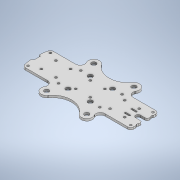
# Autodesk Inventor part: center plate
Saved by Autodesk Inventor 2020 (Build 240168000, 168)
## iProperties
Created: 2022-08-17
Part Number: center plate
Material: Generic
Document SubType Name: Modeling
Designer: Steven
Density: 1 g/cm^3
Appearance: Default
Author: Steven
Autodesk Inventor part; units mm, degrees
ref_plane "YZ Plane" through (0, 0, 0) normal (1, 0, 0) x (0, 1, 0)
ref_plane "XZ Plane" through (0, 0, 0) normal (0, 1, 0) x (-1, 0, 0)
ref_plane "XY Plane" through (0, 0, 0) normal (0, 0, 1) x (1, 0, 0)
sketch "Sketch1" plane through (0, 0, 0) normal (0, 1, 0) x (-1, 0, 0)
  arc A0 (-33.8239, -28.265) -> (-21.4136, -36.6803) centre (-27.5042, -32.3038) ccw
  line L0 (-21.4136, -36.6803) -> (-21.3077, -36.5329)
  arc A1 (21.3077, -36.5329) -> (-21.3077, -36.5329) centre (0, -51.9445) ccw
  line L1 (21.3077, -36.5329) -> (21.4136, -36.6803)
  arc A2 (21.4136, -36.6803) -> (33.8239, -28.265) centre (27.5042, -32.3038) ccw
  arc A3 (33.327, -27.1322) -> (33.8239, -28.265) centre (37.1944, -26.111) ccw
  arc A4 (39.3981, -19.25) -> (33.327, -27.1322) centre (39.3981, -25.5292) ccw
  line L2 (39.3981, -19.25) -> (69.95, -19.25)
  arc A5 (69.95, -19.25) -> (73.8582, -16.102) centre (69.95, -15.25) ccw
  arc A6 (73.8582, -16.102) -> (75.3578, -5.9597) centre (0.0002, 0) ccw
  arc A7 (75.3578, -5.9597) -> (74.448, -4.8846) centre (74.3609, -5.8808) ccw
  line L3 (74.448, -4.8846) -> (73.7452, -4.8231)
  arc A8 (72.8337, -3.7752) -> (73.7452, -4.8231) centre (73.8323, -3.8269) ccw
  arc A9 (72.8337, -3.7752) -> (72.8337, 3.7752) centre (0.0002, 0) ccw
  arc A10 (73.7452, 4.8231) -> (72.8337, 3.7752) centre (73.8323, 3.8269) ccw
  line L4 (73.7452, 4.8231) -> (74.448, 4.8846)
  arc A11 (74.448, 4.8846) -> (75.3578, 5.9597) centre (74.3609, 5.8808) ccw
  arc A12 (75.3578, 5.9597) -> (73.8582, 16.102) centre (0.0002, 0) ccw
  arc A13 (73.8582, 16.102) -> (69.95, 19.25) centre (69.95, 15.25) ccw
  line L5 (69.95, 19.25) -> (39.3981, 19.25)
  arc A14 (33.327, 27.1322) -> (39.3981, 19.25) centre (39.3981, 25.5292) ccw
  arc A15 (33.8239, 28.265) -> (33.327, 27.1322) centre (37.1944, 26.111) ccw
  arc A16 (33.8239, 28.265) -> (21.4136, 36.6803) centre (27.5042, 32.3038) ccw
  line L6 (21.4136, 36.6803) -> (21.3077, 36.5329)
  arc A17 (-21.3077, 36.5329) -> (21.3077, 36.5329) centre (0, 51.9445) ccw
  line L7 (-21.3077, 36.5329) -> (-21.4136, 36.6803)
  arc A18 (-21.4136, 36.6803) -> (-33.8239, 28.265) centre (-27.5042, 32.3038) ccw
  arc A19 (-33.327, 27.1322) -> (-33.8239, 28.265) centre (-37.1944, 26.111) ccw
  arc A20 (-39.3981, 19.25) -> (-33.327, 27.1322) centre (-39.3981, 25.5292) ccw
  line L8 (-39.3981, 19.25) -> (-70.5602, 19.25)
  arc A21 (-70.5602, 19.25) -> (-74.56, 15.2108) centre (-70.5602, 15.25) ccw
  line L9 (-74.56, 15.2108) -> (-74.56, 12.5073)
  arc A22 (-74.56, 12.5073) -> (-74.0519, 11.382) centre (-73.06, 12.5073) ccw
  arc A23 (-73.6342, 9.7438) -> (-74.0519, 11.382) centre (-75.0438, 10.2568) ccw
  line L10 (-73.6342, 9.7438) -> (-74.2404, 8.0784)
  arc A24 (-74.2404, 8.0784) -> (-74.56, 6.2657) centre (-69.26, 6.2657) ccw
  line L11 (-74.56, 6.2657) -> (-74.56, 6.25)
  arc A25 (-74.56, 6.25) -> (-71.56, 3.25) centre (-71.56, 6.25) ccw
  line L12 (-71.56, 3.25) -> (-65.309, 3.25)
  arc A26 (-65.309, -3.25) -> (-65.309, 3.25) centre (-65.309, 0) ccw
  line L13 (-65.309, -3.25) -> (-71.56, -3.25)
  arc A27 (-71.56, -3.25) -> (-74.56, -6.25) centre (-71.56, -6.25) ccw
  line L14 (-74.56, -6.25) -> (-74.56, -6.2657)
  arc A28 (-74.56, -6.2657) -> (-74.2404, -8.0784) centre (-69.26, -6.2657) ccw
  line L15 (-74.2404, -8.0784) -> (-73.6342, -9.7438)
  arc A29 (-74.0519, -11.382) -> (-73.6342, -9.7438) centre (-75.0438, -10.2568) ccw
  arc A30 (-74.0519, -11.382) -> (-74.56, -12.5073) centre (-73.06, -12.5073) ccw
  line L16 (-74.56, -12.5073) -> (-74.56, -15.2108)
  arc A31 (-74.56, -15.2108) -> (-70.5602, -19.25) centre (-70.5602, -15.25) ccw
  line L17 (-70.5602, -19.25) -> (-39.3981, -19.25)
  arc A32 (-33.327, -27.1322) -> (-39.3981, -19.25) centre (-39.3981, -25.5292) ccw
  arc A33 (-33.8239, -28.265) -> (-33.327, -27.1322) centre (-37.1944, -26.111) ccw
  circle A34 centre (-27.5042, -32.3038) radius 2.25
  arc A35 (-8.7852, -24.3068) -> (-9.9324, -22.6685) centre (-9.3588, -23.4876) ccw
  line L18 (-11.9802, -24.1024) -> (-9.9324, -22.6685)
  line L19 (58.6187, 4.75) -> (65.1187, 4.75)
  arc A36 (65.1187, 4.75) -> (65.1187, 7.75) centre (65.1187, 6.25) ccw
  line L20 (65.1187, 7.75) -> (58.6187, 7.75)
  arc A37 (58.6187, 7.75) -> (58.6187, 4.75) centre (58.6187, 6.25) ccw
  line L21 (-18.0988, -21.6995) -> (-22.3003, -27.5465)
  arc A38 (-24.6553, -25.8542) -> (-22.3003, -27.5465) centre (-23.4778, -26.7004) ccw
  circle A39 centre (27.5042, -32.3038) radius 3.15
  arc A40 (-18.0988, -21.6995) -> (-20.4538, -20.0072) centre (-19.2763, -20.8534) ccw
  line L22 (65.1187, 1.5) -> (56.2002, 1.5)
  arc A41 (56.2002, 1.5) -> (56.2002, -1.5) centre (56.2002, 0) ccw
  line L23 (56.2002, -1.5) -> (65.1187, -1.5)
  arc A42 (65.1187, -1.5) -> (65.1187, 1.5) centre (65.1187, 0) ccw
  line L24 (30.3675, -6.2794) -> (31.6059, -1.9507)
  arc A43 (33.0971, -1.3777) -> (31.6059, -1.9507) centre (32.5673, -2.2258) ccw
  line L25 (33.0971, -1.3777) -> (38.3837, -4.6803)
  arc A44 (38.0092, -6.5163) -> (38.3837, -4.6803) centre (37.8539, -5.5284) ccw
  line L26 (38.0092, -6.5163) -> (31.4843, -7.5423)
  arc A45 (30.3675, -6.2794) -> (31.4843, -7.5423) centre (31.329, -6.5544) ccw
  arc A46 (-11.9802, -24.1024) -> (-10.8331, -25.7407) centre (-11.4067, -24.9216) ccw
  circle A47 centre (-27.5042, -32.3038) radius 3.15
  line L27 (44.5187, 14.25) -> (53.5187, 14.25)
  arc A48 (53.5187, 14.25) -> (54.5187, 14.25) centre (54.0187, 14.25) ccw
  line L28 (54.5187, 14.25) -> (54.5187, 16.25)
  arc A49 (54.5187, 16.25) -> (53.5187, 16.25) centre (54.0187, 16.25) ccw
  line L29 (53.5187, 16.25) -> (44.5187, 16.25)
  arc A50 (44.5187, 16.25) -> (43.5187, 16.25) centre (44.0187, 16.25) ccw
  line L30 (43.5187, 16.25) -> (43.5187, 14.25)
  arc A51 (43.5187, 14.25) -> (44.5187, 14.25) centre (44.0187, 14.25) ccw
  line L31 (-8.7852, -24.3068) -> (-10.8331, -25.7407)
  circle A52 centre (57.0593, 10) radius 1
  arc A53 (-22.3003, 27.5465) -> (-24.6553, 25.8542) centre (-23.4778, 26.7004) ccw
  circle A54 centre (69.95, 15.25) radius 1.55
  line L32 (-9.9324, 22.6685) -> (-11.9802, 24.1024)
  line L33 (-70.7795, -9.0168) -> (-71.6345, -6.6675)
  arc A55 (-71.6345, -6.6675) -> (-72.2754, -6.3687) centre (-72.1044, -6.8386) ccw
  line L34 (-72.2754, -6.3687) -> (-72.7452, -6.5397)
  arc A56 (-72.7452, -6.5397) -> (-73.044, -7.1806) centre (-72.5742, -7.0096) ccw
  line L35 (-73.044, -7.1806) -> (-72.189, -9.5298)
  arc A57 (-72.189, -9.5298) -> (-71.5481, -9.8286) centre (-71.7192, -9.3588) ccw
  line L36 (-71.5481, -9.8286) -> (-71.0783, -9.6576)
  arc A58 (-71.0783, -9.6576) -> (-70.7795, -9.0168) centre (-71.2493, -9.1878) ccw
  circle A59 centre (-9.9998, 10) radius 1.55
  circle A60 centre (-28.2498, 15.25) radius 1.55
  arc A61 (-38.0092, 6.5163) -> (-38.3837, 4.6803) centre (-37.8539, 5.5284) ccw
  line L37 (-38.0092, 6.5163) -> (-31.4843, 7.5423)
  arc A62 (-30.3675, 6.2794) -> (-31.4843, 7.5423) centre (-31.329, 6.5544) ccw
  line L38 (-30.3675, 6.2794) -> (-31.6059, 1.9507)
  arc A63 (-33.0971, 1.3777) -> (-31.6059, 1.9507) centre (-32.5673, 2.2258) ccw
  line L39 (-33.0971, 1.3777) -> (-38.3837, 4.6803)
  line L40 (-42.405, -16.5) -> (-62.405, -16.5)
  arc A64 (-62.405, -14.5) -> (-62.405, -16.5) centre (-62.405, -15.5) ccw
  line L41 (-62.405, -14.5) -> (-42.405, -14.5)
  arc A65 (-42.405, -16.5) -> (-42.405, -14.5) centre (-42.405, -15.5) ccw
  line L42 (-71.0783, 9.6576) -> (-71.5481, 9.8286)
  arc A66 (-71.5481, 9.8286) -> (-72.189, 9.5298) centre (-71.7192, 9.3588) ccw
  line L43 (-72.189, 9.5298) -> (-73.044, 7.1806)
  arc A67 (-73.044, 7.1806) -> (-72.7452, 6.5397) centre (-72.5742, 7.0096) ccw
  line L44 (-72.7452, 6.5397) -> (-72.2754, 6.3687)
  arc A68 (-72.2754, 6.3687) -> (-71.6345, 6.6675) centre (-72.1044, 6.8386) ccw
  line L45 (-71.6345, 6.6675) -> (-70.7795, 9.0168)
  arc A69 (-70.7795, 9.0168) -> (-71.0783, 9.6576) centre (-71.2493, 9.1878) ccw
  arc A70 (-58.3158, -3.5) -> (-58.3158, -5.5) centre (-58.3158, -4.5) ccw
  line L46 (-58.3158, -5.5) -> (-52.3158, -5.5)
  arc A71 (-52.3158, -5.5) -> (-52.3158, -3.5) centre (-52.3158, -4.5) ccw
  line L47 (-52.3158, -3.5) -> (-58.3158, -3.5)
  line L48 (-10.8331, 25.7407) -> (-8.7852, 24.3068)
  arc A72 (-20.4275, 8.2673) -> (-20.8836, 6.6042) centre (-20.4038, 7.3667) ccw
  line L49 (-20.4275, 8.2673) -> (-13.542, 8.3985)
  arc A73 (-12.661, 7.2587) -> (-13.542, 8.3985) centre (-13.5284, 7.4986) ccw
  line L50 (-12.661, 7.2587) -> (-13.6696, 3.6122)
  arc A74 (-15.1632, 3.0306) -> (-13.6696, 3.6122) centre (-14.6334, 3.8788) ccw
  line L51 (-15.1632, 3.0306) -> (-20.8836, 6.6042)
  arc A75 (-20.4538, 20.0072) -> (-18.0988, 21.6995) centre (-19.2763, 20.8534) ccw
  arc A76 (-10.8331, 25.7407) -> (-11.9802, 24.1024) centre (-11.4067, 24.9216) ccw
  circle A77 centre (-57.059, 10) radius 1.55
  arc A78 (-58.3158, 5.5) -> (-58.3158, 3.5) centre (-58.3158, 4.5) ccw
  line L52 (-58.3158, 3.5) -> (-52.3158, 3.5)
  arc A79 (-52.3158, 3.5) -> (-52.3158, 5.5) centre (-52.3158, 4.5) ccw
  line L53 (-52.3158, 5.5) -> (-58.3158, 5.5)
  line L54 (-24.6553, 25.8542) -> (-20.4538, 20.0072)
  arc A80 (-9.9324, 22.6685) -> (-8.7852, 24.3068) centre (-9.3588, 23.4876) ccw
  circle A81 centre (-15.25, 15.25) radius 2.25
  line L55 (-62.405, 16.5) -> (-42.405, 16.5)
  arc A82 (-42.405, 14.5) -> (-42.405, 16.5) centre (-42.405, 15.5) ccw
  line L56 (-42.405, 14.5) -> (-62.405, 14.5)
  arc A83 (-62.405, 16.5) -> (-62.405, 14.5) centre (-62.405, 15.5) ccw
  arc A84 (-44.4091, 0.275) -> (-44.4091, -0.275) centre (-43.4477, 0) ccw
  line L57 (-44.4091, 0.275) -> (-43.6501, 2.9283)
  arc A85 (-42.1588, 3.5013) -> (-43.6501, 2.9283) centre (-42.6886, 2.6532) ccw
  line L58 (-42.1588, 3.5013) -> (-37.9117, 0.8481)
  arc A86 (-37.9117, -0.8481) -> (-37.9117, 0.8481) centre (-38.4415, 0) ccw
  line L59 (-37.9117, -0.8481) -> (-42.1588, -3.5013)
  arc A87 (-43.6501, -2.9283) -> (-42.1588, -3.5013) centre (-42.6886, -2.6532) ccw
  line L60 (-43.6501, -2.9283) -> (-44.4091, -0.275)
  arc A88 (-7.8639, 3.9177) -> (-9.3575, 3.336) centre (-8.3937, 3.0696) ccw
  line L61 (-7.8639, 3.9177) -> (-2.9502, 0.8481)
  arc A89 (-2.9502, -0.8481) -> (-2.9502, 0.8481) centre (-3.48, 0) ccw
  line L62 (-2.9502, -0.8481) -> (-7.8639, -3.9177)
  arc A90 (-9.3575, -3.336) -> (-7.8639, -3.9177) centre (-8.3937, -3.0696) ccw
  line L63 (-9.3575, -3.336) -> (-10.206, -0.2664)
  arc A91 (-10.206, 0.2664) -> (-10.206, -0.2664) centre (-9.2421, 0) ccw
  line L64 (-10.206, 0.2664) -> (-9.3575, 3.336)
  circle A92 centre (-15.25, 15.25) radius 3.15
  circle A93 centre (-37.059, 10) radius 1.55
  circle A94 centre (-70.5602, 15.25) radius 1.55
  circle A95 centre (-70.5602, -15.25) radius 1.55
  circle A96 centre (28.2502, -15.25) radius 1.55
  line L65 (22.3006, -27.5465) -> (18.0991, -21.6995)
  line L66 (10.8331, -25.7407) -> (8.7852, -24.3068)
  arc A97 (10.8331, -25.7407) -> (11.9802, -24.1024) centre (11.4067, -24.9216) ccw
  arc A98 (-0.5298, 4.0525) -> (0.5298, 4.0525) centre (0, 4.9006) ccw
  line L67 (-0.5298, 4.0525) -> (-4.9689, 6.8256)
  arc A99 (-4.4965, 8.4889) -> (-4.9689, 6.8256) centre (-4.492, 7.5889) ccw
  line L68 (-4.4965, 8.4889) -> (4.4965, 8.4889)
  arc A100 (4.9689, 6.8256) -> (4.4965, 8.4889) centre (4.492, 7.5889) ccw
  line L69 (4.9689, 6.8256) -> (0.5298, 4.0525)
  line L70 (10.206, -0.2664) -> (9.3575, -3.336)
  arc A101 (7.8639, -3.9177) -> (9.3575, -3.336) centre (8.3937, -3.0696) ccw
  line L71 (7.8639, -3.9177) -> (2.9502, -0.8481)
  arc A102 (2.9502, 0.8481) -> (2.9502, -0.8481) centre (3.48, 0) ccw
  line L72 (2.9502, 0.8481) -> (7.8639, 3.9177)
  arc A103 (9.3575, 3.336) -> (7.8639, 3.9177) centre (8.3937, 3.0696) ccw
  line L73 (9.3575, 3.336) -> (10.206, 0.2664)
  arc A104 (10.206, -0.2664) -> (10.206, 0.2664) centre (9.2421, 0) ccw
  line L74 (27.1605, 4.3044) -> (28.3132, 0.275)
  arc A105 (28.3132, -0.275) -> (28.3132, 0.275) centre (27.3517, 0) ccw
  line L75 (28.3132, -0.275) -> (27.1605, -4.3044)
  arc A106 (25.6692, -4.8775) -> (27.1605, -4.3044) centre (26.199, -4.0294) ccw
  line L76 (25.6692, -4.8775) -> (19.2192, -0.8481)
  arc A107 (19.2192, 0.8481) -> (19.2192, -0.8481) centre (19.749, 0) ccw
  line L77 (19.2192, 0.8481) -> (25.6692, 4.8775)
  arc A108 (27.1605, 4.3044) -> (25.6692, 4.8775) centre (26.199, 4.0294) ccw
  arc A109 (-4.9689, -6.8256) -> (-4.4965, -8.4889) centre (-4.492, -7.5889) ccw
  line L78 (-4.9689, -6.8256) -> (-0.5298, -4.0525)
  arc A110 (0.5298, -4.0525) -> (-0.5298, -4.0525) centre (0, -4.9006) ccw
  line L79 (0.5298, -4.0525) -> (4.9689, -6.8256)
  arc A111 (4.4965, -8.4889) -> (4.9689, -6.8256) centre (4.492, -7.5889) ccw
  line L80 (4.4965, -8.4889) -> (-4.4965, -8.4889)
  circle A112 centre (10.0002, -10) radius 1.55
  arc A113 (20.4275, -8.2673) -> (20.8836, -6.6042) centre (20.4067, -7.3675) ccw
  ellipse E0 centre (0, 0) end of major axis (87.8993, 0) minor radius 8.5 (13.542, -8.3985) -> (20.4275, -8.2673) ccw
  line L81 (12.661, -7.2587) -> (13.6696, -3.6122)
  line L82 (15.1632, -3.0306) -> (20.8836, -6.6042)
  arc A114 (13.6696, 3.6122) -> (15.1632, 3.0306) centre (14.6334, 3.8788) ccw
  arc A115 (12.661, -7.2587) -> (13.542, -8.3985) centre (13.5284, -7.4986) ccw
  arc A116 (15.1632, -3.0306) -> (13.6696, -3.6122) centre (14.6334, -3.8788) ccw
  arc A117 (20.4541, -20.0072) -> (18.0991, -21.6995) centre (19.2766, -20.8534) ccw
  arc A118 (9.9324, -22.6685) -> (8.7852, -24.3068) centre (9.3588, -23.4876) ccw
  arc A119 (22.3006, -27.5465) -> (24.6556, -25.8542) centre (23.4781, -26.7004) ccw
  circle A120 centre (15.25, -15.25) radius 2.25
  line L83 (9.9324, -22.6685) -> (11.9802, -24.1024)
  line L84 (20.4541, -20.0072) -> (24.6556, -25.8542)
  circle A121 centre (27.5042, -32.3038) radius 2.25
  circle A122 centre (37.0593, 10) radius 1
  arc A123 (44.4091, -0.275) -> (44.4091, 0.275) centre (43.4477, 0) ccw
  line L85 (44.4091, -0.275) -> (43.6501, -2.9283)
  arc A124 (42.1588, -3.5013) -> (43.6501, -2.9283) centre (42.6886, -2.6532) ccw
  line L86 (42.1588, -3.5013) -> (37.9117, -0.8481)
  arc A125 (37.9117, 0.8481) -> (37.9117, -0.8481) centre (38.4415, 0) ccw
  line L87 (37.9117, 0.8481) -> (42.1588, 3.5013)
  arc A126 (43.6501, 2.9283) -> (42.1588, 3.5013) centre (42.6886, 2.6532) ccw
  line L88 (43.6501, 2.9283) -> (44.4091, 0.275)
  line L89 (31.6059, 1.9507) -> (30.3675, 6.2794)
  arc A127 (31.4843, 7.5423) -> (30.3675, 6.2794) centre (31.329, 6.5544) ccw
  line L90 (31.4843, 7.5423) -> (38.0092, 6.5163)
  arc A128 (38.3837, 4.6803) -> (38.0092, 6.5163) centre (37.8539, 5.5284) ccw
  line L91 (38.3837, 4.6803) -> (33.0971, 1.3777)
  arc A129 (31.6059, 1.9507) -> (33.0971, 1.3777) centre (32.5673, 2.2258) ccw
  ellipse E1 centre (0, 0) end of major axis (87.8993, 0) minor radius 8.5 (20.4275, 8.2673) -> (13.542, 8.3985) ccw
  line L92 (20.8836, 6.6042) -> (15.1632, 3.0306)
  arc A130 (20.8836, 6.6042) -> (20.4275, 8.2673) centre (20.4067, 7.3675) ccw
  arc A131 (13.542, 8.3985) -> (12.661, 7.2587) centre (13.5284, 7.4986) ccw
  circle A132 centre (10.0002, 10) radius 1.55
  line L93 (13.6696, 3.6122) -> (12.661, 7.2587)
  circle A133 centre (15.25, -15.25) radius 3.15
  line L94 (24.6556, 25.8542) -> (20.4541, 20.0072)
  line L95 (43.5187, -14.25) -> (43.5187, -16.25)
  arc A134 (43.5187, -16.25) -> (44.5187, -16.25) centre (44.0187, -16.25) ccw
  line L96 (44.5187, -16.25) -> (53.5187, -16.25)
  arc A135 (53.5187, -16.25) -> (54.5187, -16.25) centre (54.0187, -16.25) ccw
  line L97 (54.5187, -16.25) -> (54.5187, -14.25)
  arc A136 (54.5187, -14.25) -> (53.5187, -14.25) centre (54.0187, -14.25) ccw
  line L98 (53.5187, -14.25) -> (44.5187, -14.25)
  arc A137 (44.5187, -14.25) -> (43.5187, -14.25) centre (44.0187, -14.25) ccw
  circle A138 centre (37.0593, -10) radius 1
  circle A139 centre (57.0593, -10) radius 1
  line L99 (58.6187, -7.75) -> (65.1187, -7.75)
  arc A140 (65.1187, -7.75) -> (65.1187, -4.75) centre (65.1187, -6.25) ccw
  line L100 (65.1187, -4.75) -> (58.6187, -4.75)
  arc A141 (58.6187, -4.75) -> (58.6187, -7.75) centre (58.6187, -6.25) ccw
  circle A142 centre (69.95, -15.25) radius 1.55
  arc A143 (8.7852, 24.3068) -> (9.9324, 22.6685) centre (9.3588, 23.4876) ccw
  arc A144 (11.9802, 24.1024) -> (10.8331, 25.7407) centre (11.4067, 24.9216) ccw
  circle A145 centre (15.25, 15.25) radius 3.15
  line L101 (11.9802, 24.1024) -> (9.9324, 22.6685)
  arc A146 (24.6556, 25.8542) -> (22.3006, 27.5465) centre (23.4781, 26.7004) ccw
  circle A147 centre (15.25, 15.25) radius 2.25
  line L102 (18.0991, 21.6995) -> (22.3006, 27.5465)
  line L103 (-18.0988, 21.6995) -> (-22.3003, 27.5465)
  line L104 (8.7852, 24.3068) -> (10.8331, 25.7407)
  circle A148 centre (28.2502, 15.25) radius 1.55
  arc A149 (18.0991, 21.6995) -> (20.4541, 20.0072) centre (19.2766, 20.8534) ccw
  arc A150 (-13.542, -8.3985) -> (-12.661, -7.2587) centre (-13.5284, -7.4986) ccw
  line L105 (-13.542, -8.3985) -> (-20.4275, -8.2673)
  arc A151 (-20.8836, -6.6042) -> (-20.4275, -8.2673) centre (-20.4067, -7.3675) ccw
  line L106 (-20.8836, -6.6042) -> (-15.1632, -3.0306)
  arc A152 (-13.6696, -3.6122) -> (-15.1632, -3.0306) centre (-14.6334, -3.8788) ccw
  line L107 (-13.6696, -3.6122) -> (-12.661, -7.2587)
  arc A153 (-19.2192, -0.8481) -> (-19.2192, 0.8481) centre (-19.749, 0) ccw
  line L108 (-19.2192, -0.8481) -> (-25.6692, -4.8775)
  arc A154 (-27.1605, -4.3044) -> (-25.6692, -4.8775) centre (-26.199, -4.0294) ccw
  line L109 (-27.1605, -4.3044) -> (-28.3132, -0.275)
  arc A155 (-28.3132, 0.275) -> (-28.3132, -0.275) centre (-27.3517, 0) ccw
  line L110 (-28.3132, 0.275) -> (-27.1605, 4.3044)
  arc A156 (-25.6692, 4.8775) -> (-27.1605, 4.3044) centre (-26.199, 4.0294) ccw
  line L111 (-25.6692, 4.8775) -> (-19.2192, 0.8481)
  circle A157 centre (-57.059, -10) radius 1.55
  circle A158 centre (-28.2498, -15.25) radius 1.55
  arc A159 (-31.6059, -1.9507) -> (-33.0971, -1.3777) centre (-32.5673, -2.2258) ccw
  line L112 (-31.6059, -1.9507) -> (-30.3675, -6.2794)
  arc A160 (-31.4843, -7.5423) -> (-30.3675, -6.2794) centre (-31.329, -6.5544) ccw
  line L113 (-31.4843, -7.5423) -> (-38.0092, -6.5163)
  arc A161 (-38.3837, -4.6803) -> (-38.0092, -6.5163) centre (-37.8539, -5.5284) ccw
  line L114 (-38.3837, -4.6803) -> (-33.0971, -1.3777)
  circle A162 centre (-15.25, -15.25) radius 2.25
  circle A163 centre (27.5042, 32.3038) radius 3.15
  circle A164 centre (27.5042, 32.3038) radius 2.25
  circle A165 centre (-27.5042, 32.3038) radius 2.25
  line L115 (-24.6553, -25.8542) -> (-20.4538, -20.0072)
  circle A166 centre (-27.5042, 32.3038) radius 3.15
  circle A167 centre (-9.9998, -10) radius 1.55
  circle A168 centre (-37.059, -10) radius 1.55
  circle A169 centre (-15.25, -15.25) radius 3.15
  point P0 (-74.0519, 11.382)
  point P1 (-74.0519, -11.382)
  point P2 (-21.4136, -36.6803)
  point P3 (21.3077, -36.5329)
  point P4 (33.8239, -28.265)
  point P5 (69.95, -19.25)
  point P6 (75.3578, -5.9597)
  point P7 (72.8337, -3.7752)
  point P8 (72.8337, 3.7752)
  point P9 (73.7452, 4.8231)
  point P10 (75.3578, 5.9597)
  point P11 (73.8582, 16.102)
  point P12 (69.95, 19.25)
  point P13 (33.327, 27.1322)
  point P14 (33.8239, 28.265)
  point P15 (-21.4136, 36.6803)
  point P16 (-33.8239, 28.265)
  point P17 (-33.327, 27.1322)
  constraints: 268 point on circle, 232 end point, 170 centre point, 8 other
extrude "fill my holes daddy" add sketch "Sketch1" along normal blind 3 contours A33 A32 L17 A31 L16 A30 A29 L15 A28 L14 A27 L13 A26 L12 A25 L11 A24 L10 A23 A22 L9 A21 L8 A20 A19 A18 L7 A17 L6 A16 A15 A14 L5 A13 A12 A11 L4 A10 A9 A8 L3 A7 A6 A5 L2 A4 A3 A2 L1 A1 L0 A0 | L31 A46 L18 A35 | A37 L20 A36 L19 | L21 A38 L115 A40 | A42 L23 A41 L22 | L24 A43 L25 A44 L26 A45 | A51 L30 A50 L29 A49 L28 A48 L27 | L103 A75 L54 A53 | L32 A76 L48 A80 | A58 L36 A57 L35 A56 L34 A55 L33 | L37 A62 L38 A63 L39 A61 | L40 A64 L41 A65 | A69 L45 A68 L44 A67 L43 A66 L42 | L49 A73 L50 A74 L51 A72 | L55 A82 L56 A83 | L57 A85 L58 A86 L59 A87 L60 A84 | L61 A89 L62 A90 L63 A91 L64 A88 | L65 A117 L84 A119 | L66 A118 L83 A97 | L67 A99 L68 A100 L69 A98 | L70 A101 L71 A102 L72 A103 L73 A104 | L74 A105 L75 A106 L76 A107 L77 A108 | L78 A110 L79 A111 L80 A109 | E0 A115 L81 A116 L82 A113 | L93 A131 E1 A130 L92 A114 | L85 A124 L86 A125 L87 A126 L88 A123 | L89 A127 L90 A128 L91 A129 | L94 A149 L102 A146 | A137 L98 A136 L97 A135 L96 A134 L95 | A141 L100 A140 L99 | L104 A144 L101 A143 | L105 A151 L106 A152 L107 A150 | L108 A154 L109 A155 L110 A156 L111 A153 | L112 A160 L113 A161 L114 A159
sketch "Sketch2" plane through (0, 0, 0) normal (0, -1, 0) x (1, 0, 0)
  circle A0 centre (-37.0593, 10) radius 1 projected
  circle A1 centre (-37.0593, -10) radius 1 projected
  circle A2 centre (-57.0593, -10) radius 1 projected
  circle A3 centre (-57.0593, 10) radius 1 projected
  circle A4 centre (-37.0593, 10) radius 1 construction
  circle A5 centre (-37.0593, -10) radius 1 construction
  line L0 (-37.0593, 10) -> (-37.0593, -10) construction
  line L1 (-37.0593, -10) -> (-37.0593, 0) construction
  circle A6 centre (-37.0593, 10) radius 1.55
  circle A7 centre (-57.0593, 10) radius 1.55
  circle A8 centre (-37.0593, -10) radius 1.55
  circle A9 centre (-57.0593, -10) radius 1.55
  point P0 (0, 0)
  dimension "d2" = 3.1
  dimension "d3" = 3.1
  dimension "d4" = 3.1
  dimension "d5" = 3.1
  constraints: 4 centre point, 4 coincident, 4 end point, 1 midpoint, 1 vertical
  measures "d2" diameter of A6
  measures "d3" diameter of A7
  measures "d4" diameter of A8
  measures "d5" diameter of A9
extrude "3m holes in the frunk" cut sketch "Sketch2" against normal through all contours A0 | A1 | A2 | A3 | A6 | A7 | A8 | A9
body "Solid1"
